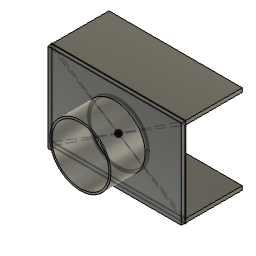
CameraControllerBox PIR adapter v0 (Autodesk Fusion 360 design; units mm, degrees)
Autodesk Fusion 360 part; units mm, degrees
sketch "Sketch1" plane through (0, 0, 0) normal (0, 1, 0) x (1, 0, 0)
  circle A0 centre (0, 0) radius 15
  line L0 (35, 21.25) -> (-35, 21.25)
  line L1 (-35, 21.25) -> (-35, -21.25)
  line L2 (-35, -21.25) -> (35, -21.25)
  line L3 (35, -21.25) -> (35, 21.25)
  line L4 (35, 21.25) -> (-35, -21.25) construction
  line L5 (-35, 21.25) -> (35, -21.25) construction
  line L6 (35, 23.25) -> (-35, 23.25)
  line L7 (-35, 23.25) -> (-35, -23.25)
  line L8 (-35, -23.25) -> (35, -23.25)
  line L9 (35, -23.25) -> (35, 23.25)
  line L10 (35, 23.25) -> (-35, -23.25) construction
  line L11 (-35, 23.25) -> (35, -23.25) construction
  circle A1 centre (0, 0) radius 16
  dimension "d1" = 30
  dimension "d2" = 70
  dimension "d3" = 42.5
  dimension "d4" = 70
  dimension "d5" = 46.5
  dimension "d6" = 32
  constraint coincident A0.centre A1.centre
  constraint horizontal L0
  constraint perpendicular L0 L1
  constraint parallel L0 L2
  constraint parallel L1 L3
  constraint coincident L4 A0.centre
  constraint coincident L5 A0.centre
  constraint horizontal L6
  constraint perpendicular L6 L7
  constraint parallel L6 L8
  constraint parallel L7 L9
  constraint coincident L10 A0.centre
  constraint coincident L11 A0.centre
  measures "d1" diameter of A0
  measures "d2" distance of L1.end L2.end
  measures "d3" distance of L0.end L1.end
  measures "d4" distance of L7.end L8.end
  measures "d5" distance of L6.end L7.end
  measures "d6" diameter of A1
extrude "Extrude1" add sketch "Sketch1" against normal blind 20 contours A1 makes body 1
extrude "Extrude2" add sketch "Sketch1" against normal blind 2 contours L0 L1 L2 L3 L7 L9 bodies 1
extrude "Extrude3" add sketch "Sketch1" along normal blind 30 separate body contours L0 L6 L7 L9 | L2 L7 L8 L9 makes body 2 at (11.6667, 10, -21.25) makes body 3 at (-11.6667, 10, 23.25)
extrude "Extrude4" add sketch "Sketch1" against normal blind 2 contours L0 L6 L7 L9 | L2 L7 L8 L9 bodies 1 2 3
equation "d4 = d2"
equation "d5 = d3 + 4 mm"
equation "d6 = d1 + 2 mm"
